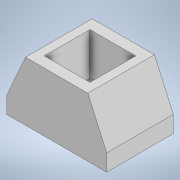
# Autodesk Inventor part: Tilt_Metal_Attachment
Saved by Autodesk Inventor 2022 (Build 260153000, 153)
## iProperties
Created: 2022-01-23
Part Number: Tilt_Metal_Attachment
Material: Generic
Document SubType Name: Modeling
Designer: Mlees
Density: 1 g/cm^3
Appearance: Default
Author: Mlees
Autodesk Inventor part; units mm, degrees
ref_plane "YZ Plane" through (0, 0, 0) normal (1, 0, 0) x (0, 1, 0)
ref_plane "XZ Plane" through (0, 0, 0) normal (0, 1, 0) x (-1, 0, 0)
ref_plane "XY Plane" through (0, 0, 0) normal (0, 0, 1) x (1, 0, 0)
sketch "Sketch1" plane through (0, 0, 0) normal (0, 1, 0) x (-1, 0, 0)
  line L0 (0, 0) -> (60, 0)
  line L1 (60, 0) -> (60, -40)
  line L2 (60, -40) -> (0, -40)
  line L3 (0, -40) -> (0, 0)
  dimension "d0" = 60
  dimension "d1" = 40
  constraints: 8 end point, 2 parallel, 1 horizontal, 1 perpendicular
  measures "d0" distance of L1.end L2.end
  measures "d1" distance of L0.end L1.end
extrude "Extrusion1" add sketch "Sketch1" along normal blind 35.4
sketch "Sketch2" plane through (0, 35.4, 0) normal (0, 1, 0) x (1, 0, 0)
  line L0 (-60, 0) -> (0, 0) projected
  line L1 (0, 40) -> (-60, 40) projected
  line L2 (-43.7, 6.3) -> (-43.7, 33.7)
  line L3 (-43.7, 33.7) -> (-16.3, 33.7)
  line L4 (-16.3, 33.7) -> (-16.3, 20)
  line L5 (-16.3, 20) -> (-16.3, 6.3)
  line L6 (-16.3, 6.3) -> (-43.7, 6.3)
  line L7 (-48.7, 38.7) -> (-48.7, 1.3)
  line L8 (-48.7, 1.3) -> (-11.3, 1.3)
  line L9 (-11.3, 1.3) -> (-11.3, 38.7)
  line L10 (-11.3, 38.7) -> (-48.7, 38.7)
  dimension "d9" = 5
  constraints: 18 end point, 7 perpendicular, 3 other
  measures "d9" distance between parallel lines of L2 L7
extrude "Extrusion2" cut sketch "Sketch2" against normal blind 25.4 contours L2 L3 L4 L5 L6
sketch "Sketch3" plane through (-60, 0, 0) normal (0, 0, 1) x (1, 0, 0)
  line L0 (60, 0) -> (60, 35.4) projected
  line L1 (60, 35.4) -> (30, 35.4)
  line L2 (0, 35.4) -> (60, 35.4) projected
  line L3 (30, 35.4) -> (11.3, 35.4)
  line L4 (0, 0) -> (0, 35.4) projected
  line L5 (0, 0) -> (0, 10)
  line L6 (0, 10) -> (11.3, 35.4)
  line L7 (0, 35.4) -> (11.3, 35.4)
  line L8 (0, 35.4) -> (0, 10)
  line L9 (60, 0) -> (0, 0) projected
  line L10 (60, 35.4) -> (0, 35.4)
  line L11 (60, 0) -> (60, 35.4)
  line L12 (60, 10) -> (48.7, 35.4)
  line L13 (60, 35.4) -> (60, 10)
  dimension "d12" = 18.7
  dimension "d13" = 10
  constraints: 20 end point, 3 point on line, 2 perpendicular, 1 midpoint
  measures "d12" distance of L1.end L3.end
  measures "d13" distance of L4.start L5.end
extrude "Extrusion3" cut sketch "Sketch3" against normal through all contours L12 L1 L0 | L4 L2 L6
sketch "Sketch4" plane through (0, 0, 0) normal (0, -1, 0) x (1, 0, 0)
  line L0 (-60, 0) -> (0, 0) projected
  line L1 (-11.3, -40) -> (-48.7, -40) projected
  circle A0 centre (-50, -10) radius 1.5
  circle A1 centre (-50, -30) radius 1.5
  circle A2 centre (-10, -30) radius 1.5
  circle A3 centre (-10, -10) radius 1.5
  dimension "d20" = 3
  constraints: 4 centre point
  measures "d20" diameter of A0
extrude "Extrusion4" cut sketch "Sketch4" against normal blind 10
body "Solid1"
